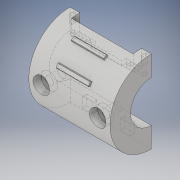
# Autodesk Inventor part: Slider Mount_B
Saved by Autodesk Inventor 2018 (Build 220112000, 112)
## iProperties
Created: 2018-01-05
Part Number: Slider Mount_B
Material: Generic
Document SubType Name: Modeling
Designer: njcfu
Density: 1 g/cm^3
Appearance: Default
Author: njcfu
Autodesk Inventor part; units mm, degrees
ref_plane "YZ Plane" through (0, 0, 0) normal (1, 0, 0) x (0, 1, 0)
sketch "Sketch2" plane through (0, 0, 0) normal (1, 0, 0) x (0, 1, 0)
  arc A0 (25.4, 0.0002) -> (-25.4, -0.0002) centre (0, 0) ccw
  arc A1 (12.7, 0.0002) -> (-12.7, 0) centre (0, 0.0002) ccw
  line L0 (-12.7, 0) -> (-25.4, -0.0002)
  line L1 (25.4, 0.0002) -> (12.7, 0.0002)
  dimension "d0" = 25.4
  dimension "d1" = 12.7
  dimension "d2" = 12.7
  dimension "d3" = 12.7
  dimension "d4" = 0.0002
  dimension "d5" = 180
  dimension "d6" = 0
  constraints: 4 end point, 4 point on circle, 2 centre point, 1 coincident, 1 horizontal
  measures "d0" radius of A0
  measures "d1" distance of L1.start L1.end
  measures "d2" distance of L0.start L0.end
  measures "d3" radius of A1
  measures "d4" distance of point (0, 0) A1.centre
  measures "d6" distance from line of A1.centre L0
extrude "Extrusion1" add sketch "Sketch2" along normal mid plane 49.9999
ref_plane "Work Plane1" through (0, 0, 25.4) normal (0, 0, 1) x (1, 0, 0)
sketch "Sketch3" plane through (0, 0, 25.4) normal (0, 0, 1) x (1, 0, 0)
  circle A0 centre (-17.38, 0) radius 5.08
  circle A1 centre (17.38, 0) radius 5.08
  line L0 (-25, 25.4) -> (-25, -25.4) projected
  line L1 (25, -25.4) -> (25, 25.4) projected
  point P0 (0, 0)
  point P1 (25, 25.4)
  dimension "d9" = 7.62
  dimension "d10" = 7.62
  dimension "d11" = 10.16
  dimension "d12" = 10.16
  dimension "d13" = 17.38
  dimension "d14" = 17.38
  constraints: 2 centre point
  measures "d9" distance from line of L0 A0.centre
  measures "d10" distance from line of L1 A1.centre
  measures "d11" diameter of A1
  measures "d12" diameter of A0
  measures "d13" distance of point (0, 0) A0.centre
  measures "d14" distance of point (0, 0) A1.centre
extrude "Extrusion2" cut sketch "Sketch3" against normal blind 5.08
sketch "Sketch4" plane through (0, 0, 0) normal (0, 0, 1) x (1, 0, 0)
  circle A0 centre (-17.38, 0) radius 2.413
  circle A1 centre (17.38, 0) radius 2.413
  line L0 (-25, 25.4) -> (-25, -25.4) projected
  line L1 (25, -25.4) -> (25, 25.4) projected
  point P0 (0, 0)
  point P1 (25, 25.4)
  dimension "d17" = 7.62
  dimension "d18" = 7.62
  dimension "d20" = 4.826
  dimension "d21" = 4.826
  dimension "d22" = 17.38
  dimension "d23" = 17.38
  constraints: 2 centre point
  measures "d17" distance from line of L0 A0.centre
  measures "d18" distance from line of L1 A1.centre
  measures "d20" diameter of A0
  measures "d21" diameter of A1
  measures "d22" distance of point (0, 0) A0.centre
  measures "d23" distance of point (0, 0) A1.centre
extrude "Extrusion3" cut sketch "Sketch4" along normal up to next
ref_plane "Work Plane2" through (0, 25.4, 0) normal (0, 1, 0) x (-1, 0, 0)
sketch "Sketch7" plane through (0, 25.4, 0) normal (0, 1, 0) x (-1, 0, 0)
  line L0 (19.05, 5.08) -> (-19.05, 5.08)
  line L1 (-19.05, 5.08) -> (-19.05, -5.08)
  line L2 (-19.05, -5.08) -> (19.05, -5.08)
  line L3 (19.05, -5.08) -> (19.05, 5.08)
  line L4 (19.05, 5.08) -> (-19.05, -5.08) construction
  line L5 (-19.05, 5.08) -> (19.05, -5.08) construction
  point P0 (0, 0)
  dimension "d33" = 38.1
  dimension "d34" = 10.16
  constraints: 12 end point, 2 midpoint, 2 parallel, 1 horizontal, 1 perpendicular
  measures "d33" distance of L1.end L2.end
  measures "d34" distance of L2.end L0.start
extrude "Extrusion5" cut sketch "Sketch7" against normal blind 10.16
sketch "Sketch8" plane through (0, 15.24, 0) normal (0, 1, 0) x (1, 0, 0)
  line L0 (9.525, 2.54) -> (-9.525, 2.54)
  line L1 (-9.525, 2.54) -> (-9.525, -2.54)
  line L2 (-9.525, -2.54) -> (9.525, -2.54)
  line L3 (9.525, -2.54) -> (9.525, 2.54)
  line L4 (9.525, 2.54) -> (-9.525, -2.54) construction
  line L5 (-9.525, 2.54) -> (9.525, -2.54) construction
  point P0 (0, 0)
  dimension "d37" = 19.05
  dimension "d38" = 5.08
  constraints: 12 end point, 2 midpoint, 2 parallel, 1 horizontal, 1 perpendicular
  measures "d37" distance of L0.start L0.end
  measures "d38" distance of L0.end L1.end
extrude "Extrusion6" cut sketch "Sketch8" against normal up to surface from surface at 0 round surface about axis through (0, 0, 0.0002) along (1, 0, 0) radius 12.7 far side no
sketch "Sketch10" plane through (25, 12.7, 0.0002) normal (0, 0, -1) x (-1, 0, 0)
  line L0 (2.54, 0.635) -> (12.7, 0.635)
  line L1 (12.7, 0.635) -> (12.7, 1.905)
  line L2 (12.7, 1.905) -> (2.54, 1.905)
  line L3 (2.54, 1.905) -> (2.54, 0.635)
  line L4 (47.4599, 0.635) -> (37.3297, 0.635)
  line L5 (37.3297, 0.635) -> (37.2999, 1.905)
  line L6 (37.2999, 1.905) -> (47.4599, 1.905)
  line L7 (47.4599, 1.905) -> (47.4599, 0.635)
  line L8 (0, 0) -> (0, 12.7) projected
  line L9 (49.9999, 12.7) -> (49.9999, 0) projected
  line L10 (49.9999, 0) -> (34.525, 0) projected
  line L11 (34.525, 2.54) -> (34.525, 0) projected
  point P0 (25, -12.7)
  dimension "d50" = 2.54
  dimension "d51" = 2.54
  dimension "d52" = 10.16
  dimension "d53" = 10.16
  dimension "d54" = 1.27
  dimension "d58" = 0.635
  dimension "d59" = 1.27
  dimension "d60" = 1.343
  constraints: 16 end point, 2 horizontal, 2 parallel, 1 perpendicular, 1 point on line
  measures "d50" distance between parallel lines of L3 L8
  measures "d51" distance between parallel lines of L9 L7
  measures "d52" distance of L1.end L2.end
  measures "d53" distance of L5.end L6.end
  measures "d54" distance of L2.end L0.start
  measures "d58" distance between parallel lines of L10 L4
  measures "d59" distance of L6.end L4.start
  measures "d60" angle of L11 L5
extrude "Extrusion8" cut sketch "Sketch10" against normal blind 2.54
sketch "Sketch12" plane through (25, 12.7, 0.0002) normal (0, 0, -1) x (-1, 0, 0)
  line L0 (3.556, 6.35) -> (2.286, 6.35)
  line L1 (2.286, 6.35) -> (2.286, 11.43)
  line L2 (2.286, 11.43) -> (3.556, 11.43)
  line L3 (3.556, 11.43) -> (3.556, 6.35)
  line L4 (3.556, 6.35) -> (2.286, 11.43) construction
  line L5 (2.286, 6.35) -> (3.556, 11.43) construction
  line L6 (46.4439, 11.43) -> (47.7139, 11.43)
  line L7 (47.7139, 11.43) -> (47.7139, 6.35)
  line L8 (47.7139, 6.35) -> (46.4439, 6.35)
  line L9 (46.4439, 6.35) -> (46.4439, 11.43)
  line L10 (46.4439, 11.43) -> (47.7139, 6.35) construction
  line L11 (47.7139, 11.43) -> (46.4439, 6.35) construction
  line L12 (0, 0) -> (0, 12.7) projected
  line L13 (0, 12.7) -> (5.95, 12.7) projected
  line L14 (49.9999, 12.7) -> (49.9999, 0) projected
  line L15 (44.05, 12.7) -> (49.9999, 12.7) projected
  point P0 (25, -12.7)
  point P1 (2.921, 8.89)
  point P2 (47.0789, 8.89)
  dimension "d74" = 2.286
  dimension "d75" = 1.27
  dimension "d76" = 1.27
  dimension "d77" = 5.08
  dimension "d78" = 1.27
  dimension "d79" = 5.08
  dimension "d80" = 2.286
  dimension "d81" = 6.35
  constraints: 24 end point, 4 midpoint, 4 parallel, 2 horizontal, 2 perpendicular
  measures "d74" distance between parallel lines of L12 L1
  measures "d75" distance of L0.start L0.end
  measures "d76" distance between parallel lines of L13 L2
  measures "d77" distance of L0.end L1.end
  measures "d78" distance of L7.end L8.end
  measures "d79" distance of L6.end L7.end
  measures "d80" distance between parallel lines of L14 L7
  measures "d81" distance between parallel lines of L15 L8
extrude "Extrusion10" cut sketch "Sketch12" against normal blind 2.54
sketch "Sketch13" plane through (0, 0, 0) normal (1, 0, 0) x (0, 1, 0)
  line L0 (0, 0) -> (12.7, 21.997)
  line L1 (11.6001, 22.632) -> (13.7999, 21.362)
  line L2 (11.6001, 22.632) -> (11.2826, 22.0821)
  line L3 (11.2826, 22.0821) -> (13.4824, 20.8121)
  line L4 (13.4824, 20.8121) -> (13.7999, 21.362)
  line L5 (11.6001, 22.632) -> (12.2351, 23.7319)
  line L6 (12.2351, 23.7319) -> (14.4349, 22.4619)
  line L7 (14.4349, 22.4619) -> (13.7999, 21.362)
  line L8 (25.4, 0.0002) -> (12.7, 0.0002) projected
  arc A0 (25.4, 0.0002) -> (-25.4, -0.0002) centre (0, 0) ccw projected
  dimension "d90" = 60
  dimension "d91" = 2.54
  dimension "d92" = 0.635
  dimension "d93" = 1.27
  dimension "d94" = 2.54
  dimension "d95" = 25.4
  dimension "d96" = 1.27
  constraints: 16 end point, 7 perpendicular, 1 point on line, 1 tangent
  measures "d90" angle of L8 L0
  measures "d91" distance of L2.end L3.end
  measures "d92" distance of L2.start L2.end
  measures "d93" distance of L1.start L5.end
  measures "d94" distance of L1.start L1.end
  measures "d95" distance of L0.start L0.end
  measures "d96" distance between parallel lines of L0 L7
extrude "Extrusion11" add sketch "Sketch13" along normal mid plane 20
fillet "Fillet2" radius 0.254 2 edges at (0, 14.4349, 22.4619) (0, 12.2351, 23.7319)
pattern_circular "Circular Pattern2" count 2 over 30 about axis through (-10, 0, 0) along (-1, 0, 0) of "Extrusion11"
fillet "Fillet3" radius 0.254 2 edges at (0, 22.4619, 14.4349) (0, 23.7319, 12.2351)
sketch "Sketch14" plane through (25, -12.7, 0) normal (0, 0.0000158, -1) x (-1, 0, 0)
  line L0 (10.16, -9.525) -> (16.51, -9.525)
  line L1 (16.51, -9.525) -> (16.51, -3.175)
  line L2 (16.51, -3.175) -> (10.16, -3.175)
  line L3 (10.16, -3.175) -> (10.16, -9.525)
  line L4 (10.16, -9.525) -> (16.51, -3.175) construction
  line L5 (16.51, -9.525) -> (10.16, -3.175) construction
  line L6 (33.4899, -9.525) -> (39.8399, -9.525)
  line L7 (39.8399, -9.525) -> (39.8399, -3.175)
  line L8 (39.8399, -3.175) -> (33.4899, -3.175)
  line L9 (33.4899, -3.175) -> (33.4899, -9.525)
  line L10 (33.4899, -9.525) -> (39.8399, -3.175) construction
  line L11 (39.8399, -9.525) -> (33.4899, -3.175) construction
  line L12 (0, -12.7) -> (0, 0) projected
  line L13 (49.9999, 0) -> (49.9999, -12.7) projected
  line L14 (49.9999, -12.7) -> (0, -12.7) projected
  point P0 (25, 12.7)
  point P1 (13.335, -6.35)
  point P2 (36.6649, -6.35)
  dimension "d104" = 10.16
  dimension "d105" = 10.16
  dimension "d106" = 6.35
  dimension "d107" = 6.35
  dimension "d108" = 3.175
  dimension "d109" = 6.35
  dimension "d110" = 6.35
  constraints: 24 end point, 4 midpoint, 4 parallel, 2 horizontal, 2 perpendicular, 1 point on line
  measures "d104" distance between parallel lines of L3 L12
  measures "d105" distance between parallel lines of L13 L7
  measures "d106" distance of L1.end L2.end
  measures "d107" distance of L0.end L1.end
  measures "d108" distance between parallel lines of L14 L0
  measures "d109" distance of L6.end L7.end
  measures "d110" distance of L7.end L8.end
extrude "Extrusion12" cut sketch "Sketch14" against normal blind 2.54
body "Solid1"
